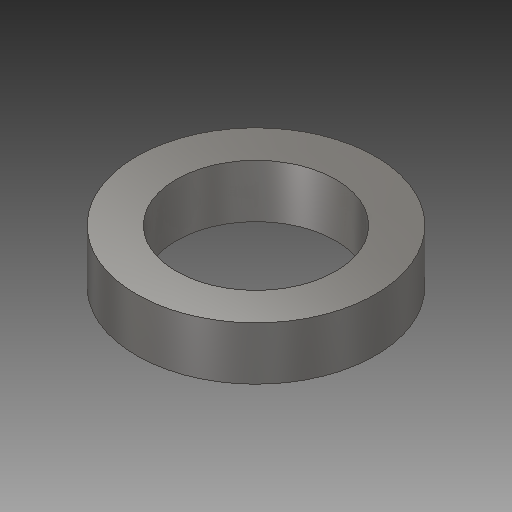
# Autodesk Inventor part: ベアリング1218.4t
Saved by Autodesk Inventor 2020 (Build 240168000, 168)
## iProperties
Part Number: ベアリング1218.4t
Material: ステンレス鋼
Document SubType Name: Modeling
Designer: 雪村
Density: 8 g/cm^3
Appearance: 半つや出し
Mass: 4.52389 g
Surface Area: 6.59734 cm^2
Volume: 0.565487 cm^3
Author: 雪村
Autodesk Inventor part; units mm, degrees
ref_plane "YZ Plane" through (0, 0, 0) normal (1, 0, 0) x (0, 1, 0)
ref_plane "XZ Plane" through (0, 0, 0) normal (0, 1, 0) x (-1, 0, 0)
ref_plane "XY Plane" through (0, 0, 0) normal (0, 0, 1) x (1, 0, 0)
sketch "スケッチ1" plane through (0, 0, 0) normal (0, 1, 0) x (-1, 0, 0)
  circle A0 centre (0, 0) radius 6
  circle A1 centre (0, 0) radius 9
  dimension "d0" = 12
  dimension "d1" = 18
  constraints: 2 centre point, 2 coincident
  measures "d0" diameter of A0
  measures "d1" diameter of A1
extrude "押し出し1" add sketch "スケッチ1" along normal blind 4
